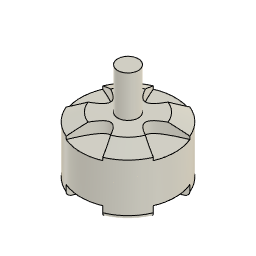
1806 v2 (Autodesk Fusion 360 design; units mm, degrees)
Autodesk Fusion 360 part; units mm, degrees
sketch "Sketch1" plane through (0, 0, 0) normal (0, 0, 1) x (1, 0, 0)
  circle A0 centre (0, 0) radius 2.5
  circle A1 centre (0, 0) radius 11.5
  line L0 (-5.6569, 5.6569) -> (5.6569, -5.6569) construction
  line L1 (4.2426, 4.2426) -> (-4.2426, -4.2426) construction
  circle A2 centre (-5.6569, 5.6569) radius 1
  circle A3 centre (4.2426, 4.2426) radius 1
  circle A4 centre (5.6569, -5.6569) radius 1
  circle A5 centre (-4.2426, -4.2426) radius 1
  line L2 (0, 0) -> (4, 0) construction
  circle A6 centre (0, 0) radius 1
  dimension "d1" = 5
  dimension "d2" = 23
  dimension "d3" = 12
  dimension "d4" = 16
  dimension "d5" = 2
  dimension "d6" = 45
  dimension "d7" = 2
  constraint coincident A0.centre A1.centre
  constraint perpendicular L0 L1
  constraint midpoint L0 L1
  constraint midpoint A0.centre L1
  constraint coincident L0.start A2.centre
  constraint coincident L1.start A3.centre
  constraint coincident L0.end A4.centre
  constraint coincident L1.end A5.centre
  constraint equal A4 A5
  constraint equal A2 A5
  constraint equal A2 A3
  constraint horizontal L2
  measures "d1" diameter of A0
  measures "d2" diameter of A1
  measures "d3" distance of L1.start L1.end
  measures "d4" distance of L0.start L0.end
  measures "d5" diameter of A3
  measures "d6" angle of L1 L2
  measures "d7" diameter of A6
extrude "Extrude1" add sketch "Sketch1" against normal blind 2 contours A6
extrude "Extrude2" add sketch "Sketch1" along normal blind 14.7 contours A0 | A1 | A2 | A3 | A4 | A5 | A6
extrude "Extrude3" add sketch "Sketch1" against normal blind 0.2 contours A0
extrude "Extrude4" cut sketch "Sketch1" along normal blind 2 contours A2 | A3 | A4 | A5
extrude "Extrude5" add sketch "Sketch1" along normal blind 24.7 contours A0 | A6
fillet "Fillet1" radius 1 1 edges at (-10.7218, -4.1586, 0)
chamfer "Chamfer1" distance 4 distance2 2 1 edges at (-10.7218, -4.1586, 14.7) measured on face at (8.4479, -0.6955, 14.7)
sketch "Sketch2" plane through (0, 0, 0) normal (0, 0, -1) x (1, 0, 0)
  circle A0 centre (0, 0) radius 2.5
  circle A1 centre (4.2426, -4.2426) radius 1
  circle A2 centre (-5.6569, -5.6569) radius 1
  circle A3 centre (5.6569, 5.6569) radius 1
  circle A4 centre (-4.2426, 4.2426) radius 1
  circle A5 centre (0, 0) radius 10.5
  spline S0 degree 2 poles (-4.4476, 10.6051) (0, 0) (4.4476, 10.6051) knots 0 0 0 1.552673 1.552673 1.552673 weights 1 1.5 1
  spline S1 degree 2 poles (-10.6051, -4.4476) (0, 0) (-10.6051, 4.4476) knots 0 0 0 1.552673 1.552673 1.552673 weights 1 1.5 1
  spline S2 degree 2 poles (4.4476, -10.6051) (0, 0) (-4.4476, -10.6051) knots 0 0 0 1.552673 1.552673 1.552673 weights 1 1.5 1
  spline S3 degree 2 poles (10.6051, 4.4476) (0, 0) (10.6051, -4.4476) knots 0 0 0 1.552673 1.552673 1.552673 weights 1 1.5 1
  circle A6 centre (0, 0) radius 11.5
  line L0 (-4.4476, 10.6051) -> (4.4476, 10.6051) construction
  dimension "d24" = 360
  constraint coincident A0.centre A5.centre
  constraint coincident S0.end A6
  constraint coincident S0.start A6
  constraint horizontal L0
extrude "Extrude6" cut sketch "Sketch2" against normal blind 2.5 contours A5 S3 | A5 S3 A6 | A5 S0 | A5 S0 A6 | A5 S2 A6 | A5 S2 | A5 S1 | A5 S1 A6
extrude "Extrude7" cut sketch "Sketch2" along normal blind -14.7 and the other way blind 12 contours A5 S3 | A5 S3 A6 | A5 S0 | A5 S0 A6 | A5 S2 A6 | A5 S2 | A5 S1 | A5 S1 A6
